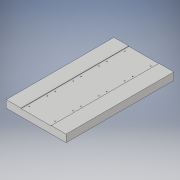
# Autodesk Inventor part: Assembly Plate
Saved by Autodesk Inventor 2019.4 (Build 234330000, 330)
## iProperties
Created: 2021-01-11
Part Number: Assembly Plate
Material: Generic
Document SubType Name: Modeling
Designer: caleb
Density: 1 g/cm^3
Appearance: Default
Author: caleb
Autodesk Inventor part; units mm, degrees
ref_plane "YZ Plane" through (0, 0, 0) normal (1, 0, 0) x (0, 1, 0)
ref_plane "XZ Plane" through (0, 0, 0) normal (0, 1, 0) x (-1, 0, 0)
ref_plane "XY Plane" through (0, 0, 0) normal (0, 0, 1) x (1, 0, 0)
sketch "Sketch1" plane through (0, 0, 0) normal (0, 1, 0) x (-1, 0, 0)
  line L0 (-60, 108) -> (60, 108)
  line L1 (60, 108) -> (60, -108)
  line L2 (60, -108) -> (-60, -108)
  line L3 (-60, -108) -> (-60, 108)
  line L4 (-60, 108) -> (60, -108) construction
  line L5 (60, 108) -> (-60, -108) construction
  point P0 (0, 0)
  dimension "d0" = 120
  dimension "d1" = 216
  constraints: 12 end point, 2 midpoint, 2 parallel, 1 horizontal, 1 perpendicular
  measures "d0" distance of L1.end L2.end
  measures "d1" distance of L0.end L1.end
extrude "Extrusion1" add sketch "Sketch1" along normal blind 14
sketch "Sketch2" plane through (0, 14, 0) normal (0, 1, 0) x (1, 0, 0)
  line L0 (-60, -108) -> (60, -108) projected
  line L1 (-60, 108) -> (-60, -108) projected
  circle A0 centre (-25.75, -95.78) radius 1.25
  circle A1 centre (-25.75, -59.68) radius 1.25
  circle A2 centre (25.75, -95.78) radius 1.25
  circle A3 centre (25.75, -59.68) radius 1.25
  circle A4 centre (-25.75, -43.96) radius 1.25
  circle A5 centre (-25.75, -7.86) radius 1.25
  circle A6 centre (25.75, -43.96) radius 1.25
  circle A7 centre (25.75, -7.86) radius 1.25
  circle A8 centre (-25.75, 7.86) radius 1.25
  circle A9 centre (-25.75, 43.96) radius 1.25
  circle A10 centre (25.75, 7.86) radius 1.25
  circle A11 centre (25.75, 43.96) radius 1.25
  circle A12 centre (-25.75, 59.68) radius 1.25
  circle A13 centre (-25.75, 95.78) radius 1.25
  circle A14 centre (25.75, 59.68) radius 1.25
  circle A15 centre (25.75, 95.78) radius 1.25
  point P0 (0, 0)
  dimension "d5" = 12.22
  dimension "d6" = 34.25
  dimension "d7" = 2.5
  dimension "d8" = 2.5
  dimension "d9" = 36.1
  dimension "d10" = 2.5
  dimension "d11" = 51.5
  dimension "d12" = 2.5
  dimension "d15" = 51.82
  constraints: 16 centre point, 2 horizontal alignment, 2 vertical alignment, 1 vertical, 24 other
  measures "d5" distance from line of L0 A0.centre
  measures "d6" distance from line of L1 A0.centre
  measures "d7" diameter of A0
  measures "d8" diameter of A1
  measures "d9" distance of A1.centre A0.centre
  measures "d10" diameter of A2
  measures "d11" distance of A2.centre A0.centre
  measures "d12" diameter of A3
  measures "d15" distance of A0.centre A4.centre
hole "Hole1" at (-25.75, 14, 95.78) at (25.75, 14, 95.78) at (25.75, 14, 59.68) at (-25.75, 14, 59.68) at (-25.75, 14, 43.96) at (25.75, 14, 43.96) at (25.75, 14, 7.86) at (-25.75, 14, 7.86) at (-25.75, 14, -7.86) at (25.75, 14, -7.86) at (25.75, 14, -43.96) at (-25.75, 14, -43.96) at (-25.75, 14, -59.68) at (25.75, 14, -59.68) at (25.75, 14, -95.78) at (-25.75, 14, -95.78) direction (0, -1, 0) diameter 1.567 end through all thread size "M2x0.4" class "6H" standard "ANSI Metric M Profile"
sketch "Sketch3" plane through (0, 14, 0) normal (0, 1, 0) x (1, 0, 0)
  line L0 (-60, -108) -> (60, -108) projected
  line L1 (60, 108) -> (-60, 108) projected
  line L2 (-60, -108) -> (-30.25, -108)
  line L3 (-30.25, -108) -> (-30.25, 108)
  line L4 (-30.25, 108) -> (-60, 108)
  line L5 (-60, 108) -> (-60, -108)
  line L6 (60, -108) -> (30.25, -108)
  line L7 (30.25, -108) -> (30.25, 108)
  line L8 (30.25, 108) -> (60, 108)
  line L9 (60, 108) -> (60, -108)
  point P0 (0, 0)
  dimension "d27" = 29.75
  dimension "d28" = 29.75
  constraints: 16 end point, 4 parallel, 2 horizontal, 2 perpendicular, 2 point on line
  measures "d27" distance between parallel lines of L5 L3
  measures "d28" distance between parallel lines of L7 L9
extrude "Extrusion2" add sketch "Sketch3" along normal blind 0.787 contours L5 L1 L3 L0 | L7 L1 L9 L0
body "Solid1"
